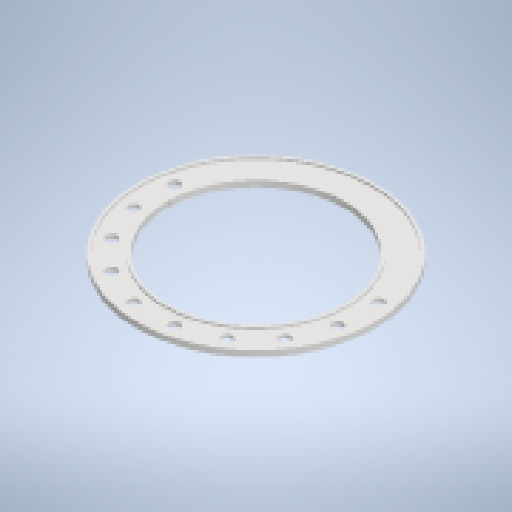
# Autodesk Inventor part: ДМС 020 кольцо прижимное 1
Saved by Autodesk Inventor 2024.2 (Build 282272000, 272)
## iProperties
Created: 2024-04-23
Part Number: ДМС 020 кольцо прижимное 1
Material: Generic
Document SubType Name: Modeling
Designer: admin
Density: 1 g/cm^3
Appearance: Default
Author: admin
Autodesk Inventor part; units mm, degrees
ref_plane "YZ Plane" through (0, 0, 0) normal (1, 0, 0) x (0, 1, 0)
ref_plane "XZ Plane" through (0, 0, 0) normal (0, 1, 0) x (-1, 0, 0)
ref_plane "XY Plane" through (0, 0, 0) normal (0, 0, 1) x (1, 0, 0)
sketch "Sketch1" plane through (0, 0, 0) normal (0, 0, 1) x (1, 0, 0)
  circle A0 centre (0, 0) radius 149
  circle A1 centre (0, 0) radius 201
  circle A2 centre (0, 0) radius 175 construction
  line L0 (0, 149) -> (0, 201) construction
  point P0 (0, 175)
  dimension "d17" = 350
  dimension "d18" = 52
  constraints: 4 vertical alignment, 3 coincident, 2 end point, 1 midpoint, 1 vertical, 6 other
  measures "d18" distance of L0.start L0.end
extrude "Extrusion1" add sketch "Sketch1" along normal blind 10
sketch "Sketch2" plane through (0, 0, 10) normal (0, 0, 1) x (1, 0, 0)
  circle A0 centre (0, 0) radius 201 construction
  circle A1 centre (0, 0) radius 149 construction
  line L0 (0, 196) -> (0, 154) construction
  line L1 (0, 149) -> (0, 0) construction
  circle A2 centre (0, 0) radius 154
  circle A3 centre (0, 0) radius 196
  circle A4 centre (0, 0) radius 175 construction
  point P0 (0, 175)
  dimension "d19" = 350
  dimension "d4" = 42
  constraints: 5 vertical alignment, 4 end point, 3 coincident, 2 vertical, 1 midpoint, 7 other
  measures "d4" distance of L0.start L0.end
extrude "Extrusion2" cut sketch "Sketch2" against normal blind 3.5
sketch "Sketch3" plane through (0, 0, 0) normal (0, 0, 1) x (1, 0, 0)
  circle A0 centre (0, 0) radius 149 construction
  circle A1 centre (0, 0) radius 201 construction
  circle A2 centre (0, 0) radius 154 projected
  circle A3 centre (0, 0) radius 196 projected
  circle A4 centre (0, 0) radius 201 projected
  line L0 (0, 0) -> (0, -201) construction
  line L1 (0, 0) -> (39.2132, -197.1378) construction
  line L2 (30.0439, -151.0409) -> (38.2377, -192.2339) construction
  circle A5 centre (34.1408, -171.6374) radius 9
  dimension "d20" = 11.25
  dimension "d21" = 18
  constraints: 6 end point, 2 point on circle, 2 point on line, 1 centre point, 1 midpoint, 1 vertical, 4 other
  measures "d20" angle of L1 L0
  measures "d21" diameter of A5
extrude "Extrusion3" cut sketch "Sketch3" along normal through all contours A5
pattern_circular "Circular Pattern2" count 10 over 202.5 about axis through (0, 0, 0) along (0, 0, -1) of "Extrusion3" both ways yes
sketch "Sketch5" plane through (0, 0, 0) normal (0, 0, -1) x (-1, 0, 0)
  circle A0 centre (0, 0) radius 149 projected
  circle A1 centre (0, 0) radius 201 projected
  line L0 (149, 0) -> (150, 0) construction
  line L1 (150, 5) -> (150, -5)
  line L2 (150, 5) -> (148.9161, 5)
  line L3 (150, -5) -> (148.9161, -5)
  line L4 (-149, 0) -> (-150, 0) construction
  line L5 (-150, 5) -> (-150, -5)
  line L6 (-150, 5) -> (-148.9161, 5)
  line L7 (-150, -5) -> (-148.9161, -5)
  dimension "d32" = 10
  dimension "d33" = 1
  constraints: 16 end point, 6 horizontal, 6 point on circle, 2 equal length, 2 horizontal alignment, 2 midpoint, 2 vertical
  measures "d32" distance of L1.start L1.end
  measures "d33" distance of L0.start L0.end
extrude "Extrusion4" cut sketch "Sketch5" against normal through all contours A0 L2 L1 L3 | A0 L7 L5 L6
equation "\"d17\" = Шпил_пласт_НОС_диам_центров"
equation "\"d19\" = Шпил_пласт_НОС_диам_центров"
equation "\"Шпил_пласт_НОС_диам_центров\" = 350"
body "Solid1"
